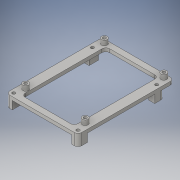
# Autodesk Inventor part: phone_clamp_v2
Saved by Autodesk Inventor 2016 (Build 200138000, 138)
## iProperties
Created: 2015-12-04
Part Number: phone_clamp_v2
Material: Generic
Document SubType Name: Modeling
Designer: jfranz
Density: 1 g/cm^3
Appearance: Default
Author: jfranz
Autodesk Inventor part; units mm, degrees
ref_plane "YZ Plane" through (0, 0, 0) normal (1, 0, 0) x (0, 1, 0)
ref_plane "XZ Plane" through (0, 0, 0) normal (0, 1, 0) x (-1, 0, 0)
ref_plane "XY Plane" through (0, 0, 0) normal (0, 0, 1) x (1, 0, 0)
sketch "Sketch8" plane through (0, 0, 0) normal (0, 1, 0) x (-1, 0, 0)
  line L0 (37.5, 50) -> (-37.5, 50)
  line L1 (-37.5, 50) -> (-37.5, -50)
  line L2 (-37.5, -50) -> (37.5, -50)
  line L3 (37.5, -50) -> (37.5, 50)
  point P0 (0, 0)
  point P1 (37.5, 0)
  point P2 (0, 50)
  dimension "d42" = 100
  dimension "d43" = 75
  constraints: 8 end point, 2 midpoint, 2 parallel, 1 horizontal, 1 horizontal alignment, 1 perpendicular, 1 vertical alignment
  measures "d42" distance of L2.end L0.start
  measures "d43" distance of L0.start L0.end
extrude "Extrusion5" add sketch "Sketch8" along normal blind 12
sketch "Sketch9" plane through (0, 12, 0) normal (0, 1, 0) x (1, 0, 0)
  line L0 (-37.5, 50) -> (-37.5, -50) projected
  line L1 (-37.5, -50) -> (37.5, -50) projected
  point P0 (0, 0)
  point P1 (-33.5, -46)
  point P2 (-33.5, 36)
  point P3 (33.5, 36)
  point P4 (33.5, -46)
  dimension "d46" = 67
  dimension "d47" = 82
  dimension "d48" = 4
  dimension "d49" = 4
  constraints: 2 horizontal alignment, 2 vertical alignment
  measures "d46" distance of point (33.5, -46) point (-33.5, -46)
  measures "d47" distance of point (-33.5, 36) point (-33.5, -46)
  measures "d48" distance from line of L0 point (-33.5, -46)
  measures "d49" distance from line of L1 point (-33.5, -46)
hole "Hole3" at (-33.5, 12, 46) at (-33.5, 12, -36) at (33.5, 12, -36) at (33.5, 12, 46) direction (0, -1, 0) diameter 3.2 end through all
sketch "Sketch10" plane through (0, 12, 0) normal (0, 1, 0) x (1, 0, 0)
  line L0 (37.5, 50) -> (-37.5, 50) projected
  point P0 (0, 0)
  point P1 (-31, -36)
  point P2 (-31, 46)
  point P3 (31, 46)
  point P4 (31, -36)
  dimension "d57" = 62
  dimension "d58" = 82
  dimension "d59" = 4
  dimension "d60" = 31
  constraints: 2 horizontal alignment, 2 vertical alignment
  measures "d57" distance of point (31, -36) point (-31, -36)
  measures "d58" distance of point (-31, -36) point (-31, 46)
  measures "d59" distance from line of L0 point (-31, 46)
  measures "d60" horizontal distance of point (-31, -36) point (0, 0)
hole "Hole4" at (-31, 12, 36) at (-31, 12, -46) at (31, 12, -46) at (31, 12, 36) direction (0, -1, 0) diameter 3.2 end through all
sketch "Sketch11" plane through (37.5, 0, 50) normal (1, 0, 0) x (0, 0, -1)
  line L0 (10, 8.5) -> (80, 8.5)
  line L1 (80, 8.5) -> (80, 0)
  line L2 (80, 0) -> (10, 0)
  line L3 (10, 0) -> (10, 8.5)
  line L4 (0, 0) -> (0, 12) projected
  line L5 (0, 0) -> (100, 0) projected
  point P0 (50, 0)
  point P1 (45, 0)
  dimension "d69" = 8.5
  dimension "d70" = 70
  dimension "d71" = 45
  constraints: 8 end point, 2 parallel, 2 point on line, 1 horizontal, 1 midpoint, 1 perpendicular
  measures "d69" distance of L2.end L0.start
  measures "d70" distance of L0.start L0.end
  measures "d71" distance from line of point (45, 0) L4
extrude "Extrusion6" cut sketch "Sketch11" against normal through all
sketch "Sketch12" plane through (-37.5, 0, 50) normal (0, 0, 1) x (1, 0, 0)
  line L0 (6.5, 8.5) -> (68.5, 8.5)
  line L1 (68.5, 8.5) -> (68.5, 0)
  line L2 (68.5, 0) -> (6.5, 0)
  line L3 (6.5, 0) -> (6.5, 8.5)
  line L4 (0, 0) -> (75, 0) projected
  point P0 (37.5, 0)
  point P1 (37.5, 0)
  dimension "d74" = 8.5
  dimension "d75" = 62
  constraints: 8 end point, 2 midpoint, 2 parallel, 1 horizontal, 1 perpendicular
  measures "d74" distance of L2.end L0.start
  measures "d75" distance of L0.start L0.end
extrude "Extrusion7" cut sketch "Sketch12" against normal through all
sketch "Sketch13" plane through (37.5, 0, -50) normal (1, 0, 0) x (0, 0, -1)
  line L0 (0, 0) -> (0, 12) projected
  line L1 (0, 0) -> (-10, 0)
  line L2 (-10, 0) -> (-10, 8.5)
  line L3 (-10, 8.5) -> (0, 8.5)
  line L4 (0, 8.5) -> (0, 0)
  line L5 (-20, 8.5) -> (-20, 0) projected
  line L6 (-90, 8.5) -> (-20, 8.5) projected
  point P0 (-50, 0)
  dimension "d78" = 10
  constraints: 8 end point, 2 parallel, 1 collinear, 1 horizontal, 1 perpendicular
  measures "d78" distance between parallel lines of L5 L2
extrude "Extrusion8" cut sketch "Sketch13" against normal through all
fillet "Fillet1" radius 4 6 edges at (-37.5, 4.25, -40) (-37.5, 10.25, -50) (-37.5, 6, 50) (37.5, 6, 50) (37.5, 4.25, -40) (37.5, 10.25, -50)
sketch "Sketch14" plane through (0, 12, 0) normal (0, 1, 0) x (1, 0, 0)
  line L0 (-23.5, -44) -> (23.5, -44)
  line L1 (27.5, -40) -> (27.5, 40)
  line L2 (23.5, 44) -> (-23.5, 44)
  line L3 (-27.5, 40) -> (-27.5, -40)
  line L4 (-33.5, -50) -> (33.5, -50) projected
  line L5 (33.5, 50) -> (-33.5, 50) projected
  line L6 (-37.5, 46) -> (-37.5, -46) projected
  line L7 (37.5, -46) -> (37.5, 46) projected
  arc A0 (-27.5, -40) -> (-23.5, -44) centre (-23.5, -40) ccw
  arc A1 (23.5, -44) -> (27.5, -40) centre (23.5, -40) ccw
  arc A2 (27.5, 40) -> (23.5, 44) centre (23.5, 40) ccw
  arc A3 (-23.5, 44) -> (-27.5, 40) centre (-23.5, 40) ccw
  point P0 (0, 0)
  dimension "d82" = 6
  dimension "d83" = 6
  dimension "d84" = 10
  dimension "d85" = 10
  dimension "d86" = 4
  constraints: 8 end point, 8 point on circle, 8 tangent, 4 centre point, 3 equal radius, 2 parallel, 1 horizontal, 1 perpendicular
  measures "d82" distance between parallel lines of L4 L0
  measures "d83" distance between parallel lines of L5 L2
  measures "d84" distance between parallel lines of L6 L3
  measures "d85" distance between parallel lines of L7 L1
  measures "d86" radius of A0
extrude "Extrusion9" cut sketch "Sketch14" against normal through all
sketch "Sketch15" plane through (0, 12, 0) normal (0, 1, 0) x (1, 0, 0)
  circle A0 centre (-31, 46) radius 1.6 projected
  circle A1 centre (-31, 46) radius 3
  circle A2 centre (-31, -36) radius 1.6 projected
  circle A3 centre (-31, -36) radius 3
  circle A4 centre (31, -36) radius 1.6 projected
  circle A5 centre (31, -36) radius 3
  circle A6 centre (31, 46) radius 1.6 projected
  circle A7 centre (31, 46) radius 3
  point P0 (0, 0)
  dimension "d89" = 6
  dimension "d90" = 6
  dimension "d91" = 6
  dimension "d92" = 6
  constraints: 4 centre point, 4 coincident
  measures "d89" diameter of A1
  measures "d90" diameter of A3
  measures "d91" diameter of A7
  measures "d92" diameter of A5
extrude "Extrusion10" add sketch "Sketch15" along normal blind 5
sketch "Sketch16" plane through (37.5, 8.5, -30) normal (0, -1, 0) x (1, 0, 0)
  circle A0 centre (-6.5, 66) radius 1.6 projected
  circle A1 centre (-6.5, 66) radius 3 projected
  line L0 (-6.5, 63) -> (-9.0981, 64.5)
  line L1 (-9.0981, 64.5) -> (-9.0981, 67.5)
  line L2 (-9.0981, 67.5) -> (-6.5, 69)
  line L3 (-6.5, 69) -> (-3.9019, 67.5)
  line L4 (-3.9019, 67.5) -> (-3.9019, 64.5)
  line L5 (-3.9019, 64.5) -> (-6.5, 63)
  circle A2 centre (-68.5, -16) radius 1.6 projected
  circle A3 centre (-68.5, -16) radius 3 projected
  line L6 (-68.5, -13) -> (-65.9019, -14.5)
  line L7 (-65.9019, -14.5) -> (-65.9019, -17.5)
  line L8 (-65.9019, -17.5) -> (-68.5, -19)
  line L9 (-68.5, -19) -> (-71.0981, -17.5)
  line L10 (-71.0981, -17.5) -> (-71.0981, -14.5)
  line L11 (-71.0981, -14.5) -> (-68.5, -13)
  circle A4 centre (-68.5, 66) radius 1.6 projected
  circle A5 centre (-68.5, 66) radius 3 projected
  line L12 (-68.5, 63) -> (-71.0981, 64.5)
  line L13 (-71.0981, 64.5) -> (-71.0981, 67.5)
  line L14 (-71.0981, 67.5) -> (-68.5, 69)
  line L15 (-68.5, 69) -> (-65.9019, 67.5)
  line L16 (-65.9019, 67.5) -> (-65.9019, 64.5)
  line L17 (-65.9019, 64.5) -> (-68.5, 63)
  circle A6 centre (-6.5, -16) radius 3 projected
  line L18 (-6.5, -19) -> (-9.0981, -17.5)
  line L19 (-9.0981, -17.5) -> (-9.0981, -14.5)
  line L20 (-9.0981, -14.5) -> (-6.5, -13)
  line L21 (-6.5, -13) -> (-3.9019, -14.5)
  line L22 (-3.9019, -14.5) -> (-3.9019, -17.5)
  line L23 (-3.9019, -17.5) -> (-6.5, -19)
  point P0 (-37.5, 30)
  point P1 (-6.5, -16)
  constraints: 48 end point, 4 vertical alignment, 3 coincident, 56 other
extrude "Extrusion11" cut sketch "Sketch16" against normal blind 3 contours L4 L5 L0 L1 L2 L3 | L7 L8 L9 L10 L11 L6 | A4 | L16 L17 L12 L13 L14 L15 | L22 L23 L18 L19 L20 L21
equation "\"d60\" = 0.5 * d57"
equation "\"d83\" = d82"
equation "\"d85\" = d84"
equation "\"d90\" = d89"
equation "\"d91\" = d89"
equation "\"d92\" = d89"
body "Solid2"
